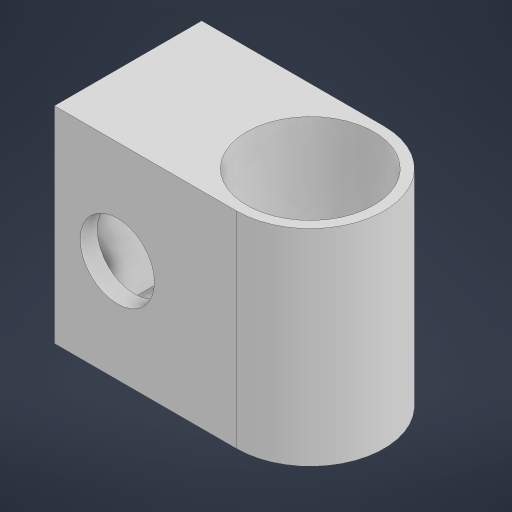
# Autodesk Inventor part: schimbator_support
Saved by Autodesk Inventor 2023 (Build 270158000, 158)
## iProperties
Created: 2022-09-22
Part Number: schimbator_support
Material: Generic
Document SubType Name: Modeling
Designer: CB110-09
Density: 1 g/cm^3
Appearance: Default
Author: CB110-09
Autodesk Inventor part; units mm, degrees
ref_plane "YZ Plane" through (0, 0, 0) normal (1, 0, 0) x (0, 1, 0)
ref_plane "XZ Plane" through (0, 0, 0) normal (0, 1, 0) x (-1, 0, 0)
ref_plane "XY Plane" through (0, 0, 0) normal (0, 0, 1) x (1, 0, 0)
sketch "Sketch1" plane through (0, 0, 0) normal (0, 1, 0) x (-1, 0, 0)
  circle A0 centre (0, 0) radius 11.125
  circle A1 centre (0, 0) radius 12.875
  line L0 (0, 12.875) -> (12.875, 12.875)
  line L1 (0, -12.875) -> (12.875, -12.875)
  line L2 (12.875, 0) -> (12.875, 12.875)
  line L3 (12.875, 0) -> (12.875, -12.875)
  dimension "d0" = 22.25
  dimension "d1" = 25.75
  constraints: 8 end point, 3 point on circle, 2 centre point, 2 coincident, 2 horizontal, 1 perpendicular, 1 point on line, 1 tangent
  measures "d0" diameter of A0
  measures "d1" diameter of A1
extrude "Extrusion1" add sketch "Sketch1" along normal blind 36
sketch "Sketch2" plane through (-12.875, 0, -12.875) normal (-1, 0, 0) x (0, 0, 1)
  line L0 (0.2295, 33) -> (25.75, 33)
  line L1 (25.75, 0) -> (25.75, 36) projected
  line L2 (25.75, 3) -> (0, 3)
  line L3 (0, 0) -> (0, 36) projected
  line L4 (0, 0) -> (25.75, 0) projected
  line L5 (0, 36) -> (25.75, 36) projected
  line L6 (22.75, 36) -> (22.75, 0)
  line L7 (0, 33) -> (0.2295, 33)
  point P0 (12.875, 0)
  point P1 (12.875, 3)
  point P2 (12.875, 0)
  point P3 (12.875, 36)
  point P4 (12.9897, 33)
  point P5 (22.75, 33)
  point P6 (22.75, 3)
  dimension "d4" = 3
  dimension "d5" = 3
  dimension "d6" = 3
  constraints: 8 end point, 6 point on line, 4 midpoint, 2 horizontal, 1 parallel, 1 perpendicular
  measures "d4" distance of point (12.875, 3) point (12.875, 0)
  measures "d5" vertical distance of point (12.875, 36) point (12.99, 33)
  measures "d6" distance between parallel lines of L1 L6
extrude "Extrusion2" add sketch "Sketch2" along normal blind 16 contours L7 L3 L5 L6 L0 | L6 L5 L1 L0 | L0 L1 L2 L6 | L6 L4 L3 L2 | L2 L1 L4 L6
sketch "Sketch3" plane through (-28.875, 0, -12.875) normal (-1, 0, 0) x (0, 0, 1)
  line L0 (25.75, 0) -> (25.75, 36) projected
  line L1 (0, 36) -> (25.75, 36)
  line L2 (25.75, 36) -> (25.75, 0)
  line L3 (25.75, 0) -> (0, 0)
  line L4 (0, 0) -> (0, 36)
  point P0 (12.875, 0)
  constraints: 8 end point, 2 parallel, 1 horizontal, 1 perpendicular
extrude "Extrusion3" add sketch "Sketch3" along normal blind 3
sketch "Sketch4" plane through (-12.875, 3, 9.875) normal (0, 0, -1) x (-1, 0, 0)
  line L0 (16, 30) -> (16, 0) projected
  line L1 (0, 30) -> (16, 30)
  line L2 (16, 30) -> (16, 0)
  line L3 (16, 0) -> (0, 0)
  line L4 (0, 0) -> (0, 30)
  line L5 (0, 30) -> (16, 0)
  line L6 (0, 0) -> (16, 30)
  circle A0 centre (8, 15) radius 6.5
  point P0 (-12.875, -3)
  dimension "d11" = 13
  constraints: 12 end point, 2 parallel, 1 centre point, 1 horizontal, 1 midpoint, 1 perpendicular
  measures "d11" diameter of A0
extrude "Extrusion4" cut sketch "Sketch4" against normal blind 3 contours A0 L5 L6 | L6 L5 A0 | A0 L6 L5 | L5 L6 A0
body "Solid1"
